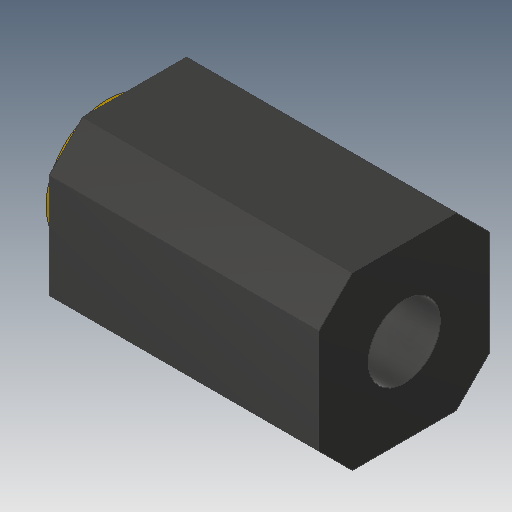
# Autodesk Inventor part: body
Saved by Autodesk Inventor 2018 (Build 220112000, 112)
## iProperties
Created: 2016-05-20
Part Number: body
Material: ABS Plastic
Document SubType Name: Modeling
Designer: Jonathan
Density: 1.06 g/cm^3
Appearance: Smooth - Black
Author: Jonathan
Autodesk Inventor part; units mm, degrees
ref_plane "YZ Plane" through (0, 0, 0) normal (1, 0, 0) x (0, 1, 0)
ref_plane "XZ Plane" through (0, 0, 0) normal (0, 1, 0) x (-1, 0, 0)
ref_plane "XY Plane" through (0, 0, 0) normal (0, 0, 1) x (1, 0, 0)
sketch "Sketch1" plane through (0, 0, 0) normal (1, 0, 0) x (0, 1, 0)
  line L0 (1.27, 1.27) -> (-1.27, 1.27)
  line L1 (-1.27, 1.27) -> (-1.27, -1.27)
  line L2 (-1.27, -1.27) -> (1.27, -1.27)
  line L3 (1.27, -1.27) -> (1.27, 1.27)
  point P0 (0, 0)
  point P1 (0, 1.27)
  point P2 (1.27, 0)
  dimension "d0" = 2.54
  dimension "d1" = 2.54
  constraints: 8 end point, 2 midpoint, 2 parallel, 1 horizontal, 1 horizontal alignment, 1 perpendicular, 1 vertical alignment
  measures "d0" distance of L2.end L0.start
  measures "d1" distance of L1.end L2.end
extrude "Extrusion1" add sketch "Sketch1" along normal blind 4
sketch "Sketch2" plane through (0, 0, 0) normal (-1, 0, 0) x (0, 0, 1)
  circle A0 centre (0, 0) radius 0.915
  dimension "d4" = 1.83
  constraints: 1 centre point, 1 coincident
  measures "d4" diameter of A0
extrude "Extrusion2" add sketch "Sketch2" along normal blind 0.4 separate body
sketch "Sketch3" plane through (4, 0, 0) normal (1, 0, 0) x (0, 0, -1)
  circle A0 centre (0, 0) radius 0.535
  dimension "d7" = 1.07
  constraints: 1 centre point, 1 coincident
  measures "d7" diameter of A0
extrude "Extrusion3" cut sketch "Sketch3" against normal blind 4 bodies 1
chamfer "Chamfer1" distance 0.5 angle 45 4 edges at (2, 1.27, -1.27) (2, -1.27, 1.27) (2, 1.27, 1.27) (2, -1.27, -1.27)
body "Solid1"
body "Solid2"
